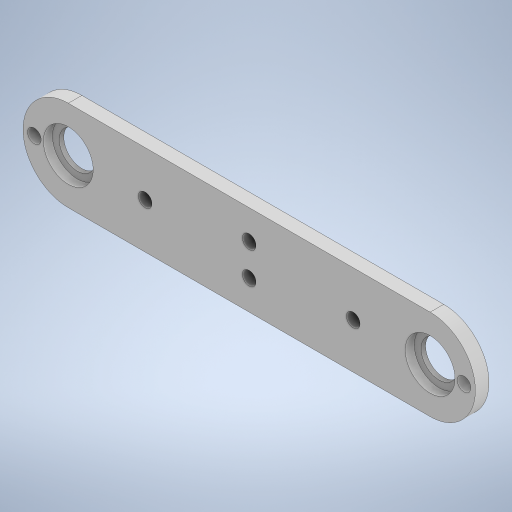
# Autodesk Inventor part: Arm4
Saved by Autodesk Inventor 2023 (Build 270158000, 158)
## iProperties
Created: 2024-02-06
Part Number: Arm4
Material: Generic
Document SubType Name: Modeling
Designer: victo
Density: 1 g/cm^3
Appearance: Default
Author: victo
Autodesk Inventor part; units mm, degrees
ref_plane "YZ Plane" through (0, 0, 0) normal (1, 0, 0) x (0, 1, 0)
ref_plane "XZ Plane" through (0, 0, 0) normal (0, 1, 0) x (-1, 0, 0)
ref_plane "XY Plane" through (0, 0, 0) normal (0, 0, 1) x (1, 0, 0)
sketch "Sketch1" plane through (0, 0, 0) normal (0, 0, 1) x (1, 0, 0)
  line L0 (0, 0) -> (80, 0) construction
  line L1 (0, -10) -> (80, -10)
  line L2 (80, 10) -> (0, 10)
  arc A0 (0, 10) -> (0, -10) centre (0, 0) ccw
  arc A1 (80, -10) -> (80, 10) centre (80, 0) ccw
  line L3 (0, 0) -> (80, 0) construction
  circle A2 centre (0, 0) radius 4
  circle A3 centre (80, 0) radius 4
  circle A4 centre (40, 3.5) radius 1.5
  circle A5 centre (40, -3.5) radius 1.5
  circle A6 centre (87.5, 0) radius 1.5
  circle A7 centre (-7.5, 0) radius 1.5
  circle A8 centre (17, 0) radius 1.5
  circle A9 centre (63, 0) radius 1.5
  point P0 (40, 0)
  point P1 (40, 0)
  dimension "d0" = 80
  dimension "d1" = 0
  dimension "d2" = 20
  dimension "d3" = 8
  dimension "d4" = 8
  dimension "d5" = 3
  dimension "d6" = 3
  dimension "d7" = 3
  dimension "d8" = 3
  dimension "d9" = 0
  dimension "d10" = 7.5
  dimension "d11" = 0
  dimension "d12" = 7.5
  dimension "d13" = 3
  dimension "d14" = 3
  dimension "d15" = 3.5
  dimension "d16" = 3.5
  dimension "d17" = 17
  dimension "d18" = 17
  dimension "d19" = 0
  dimension "d20" = 0
  constraints: 10 centre point, 10 end point, 4 point on circle, 4 tangent, 2 coincident, 2 horizontal, 2 midpoint, 2 point on line, 1 collinear, 1 parallel
  measures "d0" distance of L0.start L0.end
  measures "d1" distance between parallel lines of L0 L3
  measures "d2" diameter of A1
  measures "d3" diameter of A2
  measures "d4" diameter of A3
  measures "d5" diameter of A4
  measures "d6" diameter of A5
  measures "d7" diameter of A6
  measures "d8" diameter of A7
  measures "d9" distance from line of L0 A6.centre
  measures "d10" distance of L0.end A6.centre
  measures "d11" distance from line of L0 A7.centre
  measures "d12" distance of L0.start A7.centre
  measures "d13" diameter of A8
  measures "d14" diameter of A9
  measures "d15" distance of point (40, 0) A4.centre
  measures "d16" distance of A5.centre point (40, 0)
  measures "d17" distance of A9.centre L0.end
  measures "d18" distance of L0.start A8.centre
  measures "d19" horizontal distance of A4.centre point (40, 0)
  measures "d20" horizontal distance of point (40, 0) A5.centre
extrude "Extrusion1" add sketch "Sketch1" along normal blind 3
sketch "Sketch2" plane through (0, 0, 3) normal (0, 0, 1) x (1, 0, 0)
  circle A0 centre (0, 0) radius 4 projected
  circle A1 centre (80, 0) radius 4 projected
  circle A2 centre (0, 0) radius 5.5
  circle A3 centre (80, 0) radius 5.5
  dimension "d23" = 11
  dimension "d24" = 11
  constraints: 2 centre point, 2 coincident
  measures "d23" diameter of A2
  measures "d24" diameter of A3
extrude "Extrusion2" cut sketch "Sketch2" against normal blind 2 contours A0 | A1 | A2 | A3
body "Solid1"
